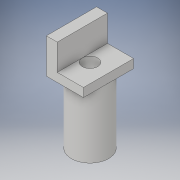
# Autodesk Inventor part: CajonInf
Saved by Autodesk Inventor 2019 (Build 230136000, 136)
## iProperties
Created: 2020-08-08
Part Number: CajonInf
Material: Generic
Document SubType Name: Modeling
Designer: Sergio
Density: 1 g/cm^3
Appearance: Default
Author: Sergio
Autodesk Inventor part; units mm, degrees
ref_plane "YZ Plane" through (0, 0, 0) normal (1, 0, 0) x (0, 1, 0)
ref_plane "XZ Plane" through (0, 0, 0) normal (0, 1, 0) x (-1, 0, 0)
ref_plane "XY Plane" through (0, 0, 0) normal (0, 0, 1) x (1, 0, 0)
sketch "Sketch1" plane through (0, 0, 0) normal (0, 1, 0) x (-1, 0, 0)
  circle A0 centre (0, 0) radius 4.25
  circle A1 centre (0, 0) radius 1.75
  dimension "d0" = 8.5
  dimension "d1" = 3.5
  constraints: 2 centre point, 2 coincident
  measures "d0" diameter of A0
  measures "d1" diameter of A1
extrude "Extrusion1" add sketch "Sketch1" along normal blind 15
sketch "Sketch2" plane through (0, 15, 0) normal (0, 1, 0) x (1, 0, 0)
  line L0 (4.25, 3.75) -> (-4.25, 3.75) construction
  line L1 (-4.25, 3.75) -> (-4.25, -3.75) construction
  line L2 (-4.25, -3.75) -> (4.25, -3.75) construction
  line L3 (4.25, -3.75) -> (4.25, 3.75) construction
  line L4 (4.25, 3.75) -> (-4.25, -3.75) construction
  line L5 (-4.25, 3.75) -> (4.25, -3.75) construction
  line L6 (-4.25, -5.75) -> (4.25, -5.75)
  line L7 (4.25, -5.75) -> (4.25, 5.75)
  line L8 (4.25, 5.75) -> (-4.25, 5.75)
  line L9 (-4.25, 5.75) -> (-4.25, -5.75)
  circle A0 centre (0, 0) radius 1.75
  circle A1 centre (0, 0) radius 1.75 projected
  dimension "d4" = 8.5
  dimension "d5" = 7.5
  dimension "d6" = 11.5
  dimension "d7" = 5.75
  constraints: 20 end point, 4 parallel, 2 collinear, 2 concentric, 2 horizontal, 2 midpoint, 2 perpendicular, 1 centre point
  measures "d4" distance of L2.end L1.end
  measures "d5" distance of L1.end L0.end
  measures "d6" distance between parallel lines of L8 L6
  measures "d7" distance from line of point (0, 0) L8
extrude "Extrusion2" add sketch "Sketch2" along normal blind 2
sketch "Sketch3" plane through (0, 17, 0) normal (0, 1, 0) x (1, 0, 0)
  line L0 (-4.25, -5.75) -> (4.25, -5.75) projected
  line L1 (4.25, 5.75) -> (-4.25, 5.75) projected
  line L2 (-4.25, -5.75) -> (-1.75, -5.75)
  line L3 (-1.75, -5.75) -> (-1.75, 5.75)
  line L4 (-1.75, 5.75) -> (-4.25, 5.75)
  line L5 (-4.25, 5.75) -> (-4.25, -5.75)
  point P0 (0, 0)
  dimension "d10" = 2.5
  constraints: 8 end point, 2 parallel, 1 horizontal, 1 perpendicular, 1 point on line
  measures "d10" distance between parallel lines of L3 L5
extrude "Extrusion3" add sketch "Sketch3" along normal blind 6
body "Solid1"
